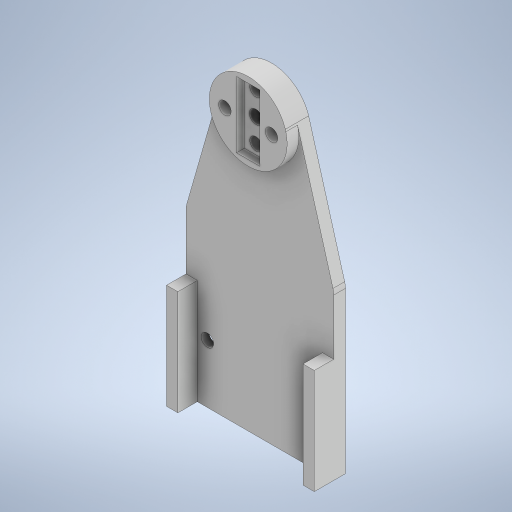
# Autodesk Inventor part: robot-arm-frame-output
Saved by Autodesk Inventor 2024.3 (Build 283343000, 343)
## iProperties
Created: 2024-11-17
Part Number: robot-arm-frame-output
Material: 一般
Document SubType Name: Modeling
Designer: azara
Density: 1 g/cm^3
Appearance: 既定
Author: azara
Autodesk Inventor part; units mm, degrees
ref_plane "YZ Plane" through (0, 0, 0) normal (1, 0, 0) x (0, 1, 0)
ref_plane "XZ Plane" through (0, 0, 0) normal (0, 1, 0) x (-1, 0, 0)
ref_plane "XY Plane" through (0, 0, 0) normal (0, 0, 1) x (1, 0, 0)
sketch "スケッチ1" plane through (0, 0, 0) normal (0, 0, 1) x (1, 0, 0)
  line L0 (0, 0) -> (38, 0)
  line L1 (38, 0) -> (38, 42)
  line L2 (38, 42) -> (0, 42)
  line L3 (0, 42) -> (0, 0)
  line L4 (19, 42) -> (19, 72)
  circle A0 centre (19, 72) radius 10
  line L5 (9.4606, 75) -> (28.5394, 75)
  line L6 (9.4606, 75) -> (0, 42)
  line L7 (28.5394, 75) -> (38, 42)
  dimension "d0" = 42
  dimension "d1" = 38
  dimension "d2" = 30
  dimension "d3" = 20
  dimension "d4" = 3
  constraints: 16 end point, 2 horizontal, 2 parallel, 2 point on circle, 1 centre point, 1 coincident, 1 midpoint, 1 perpendicular, 1 vertical
  measures "d0" distance of L0.end L1.end
  measures "d1" distance of L0.start L0.end
  measures "d2" distance of L4.start L4.end
  measures "d3" diameter of A0
  measures "d4" distance from line of L4.end L5
extrude "押し出し1" add sketch "スケッチ1" along normal blind 3
sketch "スケッチ2" plane through (0, 0, 3) normal (0, 0, 1) x (1, 0, 0)
  line L0 (0, 0) -> (38, 0) projected
  line L1 (38, 0) -> (38, 42) projected
  line L2 (38, 42) -> (28.5394, 75) projected
  arc A0 (28.5394, 75) -> (9.4606, 75) centre (19, 72) ccw projected
  circle A1 centre (19, 72) radius 10
  point P0 (9.4606, 75)
  point P1 (28.6799, 74.5099)
  constraints: 1 coincident, 3 other
extrude "押し出し2" add sketch "スケッチ2" along normal blind 3
sketch "スケッチ4" plane through (0, 0, 3) normal (0, 0, 1) x (1, 0, 0)
  line L0 (0, 42) -> (0, 0) projected
  line L1 (0, 0) -> (2.9, 0)
  line L2 (2.9, 0) -> (2.9, 27)
  line L3 (2.9, 27) -> (0, 27)
  line L4 (0, 27) -> (0, 0)
  line L5 (0, 0) -> (38, 0) projected
  line L6 (38, 0) -> (35.1, 0)
  line L7 (35.1, 0) -> (35.1, 27)
  line L8 (35.1, 27) -> (38, 27)
  line L9 (38, 27) -> (38, 0)
  point P0 (0, 27)
  dimension "d32" = 2.9
  dimension "d33" = 2.9
  dimension "d34" = 27
  dimension "d35" = 27
  constraints: 16 end point, 4 parallel, 2 horizontal, 2 perpendicular
  measures "d32" distance of L2.end L3.end
  measures "d33" distance of L7.end L8.end
  measures "d34" distance of L8.end L5.end
  measures "d35" distance of L1.end L2.end
extrude "押し出し3" add sketch "スケッチ4" along normal blind 5
sketch "スケッチ5" plane through (0, 0, 3) normal (0, 0, 1) x (1, 0, 0)
  line L0 (2.9, 0) -> (35.1, 0) projected
  line L1 (35.1, 27) -> (35.1, 0) projected
  point P0 (0, 0)
  point P1 (5.5, 15)
  point P2 (32.5, 15)
  dimension "d38" = 15
  dimension "d39" = 15
  dimension "d40" = 2.6
  dimension "d41" = 27
  measures "d38" distance from line of L0 point (32.5, 15)
  measures "d39" distance from line of L0 point (5.5, 15)
  measures "d40" distance from line of L1 point (32.5, 15)
  measures "d41" distance of point (32.5, 15) point (5.5, 15)
hole "穴2" at (5.5, 15, 3) at (32.5, 15, 3) direction (0, 0, -1) diameter 3.2 end through all
sketch "スケッチ7" plane through (0, 0, 0) normal (0, 0, -1) x (-1, 0, 0)
  circle A0 centre (-32.5, 15) radius 1.6 projected
  circle A1 centre (-32.5, 15) radius 4
  circle A2 centre (-5.5, 15) radius 1.6 projected
  circle A3 centre (-5.5, 15) radius 4
  point P0 (0, 0)
  dimension "d58" = 8
  dimension "d59" = 8
  constraints: 4 coincident, 2 centre point
  measures "d58" diameter of A1
  measures "d59" diameter of A3
extrude "押し出し4" cut sketch "スケッチ7" against normal blind 1
sketch "スケッチ8" plane through (0, 0, 0) normal (0, 0, -1) x (-1, 0, 0)
  circle A0 centre (-5.5, 15) radius 4 projected
  circle A1 centre (-32.5, 15) radius 4 projected
  line L0 (0, 42) -> (0, 0) projected
  line L1 (-9.4606, 75) -> (0, 42) projected
  arc A2 (-9.4606, 75) -> (-28.5394, 75) centre (-19, 72) ccw projected
  line L2 (-38, 42) -> (-28.5394, 75) projected
  line L3 (-38, 0) -> (-38, 42) projected
  line L4 (0, 0) -> (-38, 0) projected
  point P0 (-19, 78)
  point P1 (-25, 72)
  point P2 (-19, 66)
  point P3 (-13, 72)
  dimension "d62" = 6
  dimension "d65" = 360
  constraints: 5 other
  measures "d62" distance of A2.centre point (-19, 78)
hole "穴4" at (19, 78, 0) at (25, 72, 0) at (19, 66, 0) at (13, 72, 0) direction (0, 0, 1) diameter 3.2 end through all
sketch "スケッチ9" plane through (0, 0, 0) normal (0, 0, -1) x (-1, 0, 0)
  circle A0 centre (-13, 72) radius 1.6 projected
  circle A1 centre (-19, 66) radius 1.6 projected
  circle A2 centre (-25, 72) radius 1.6 projected
  circle A3 centre (-19, 78) radius 1.6 projected
  circle A4 centre (-5.5, 15) radius 4 projected
  circle A5 centre (-32.5, 15) radius 4 projected
  line L0 (0, 42) -> (0, 0) projected
  line L1 (-9.4606, 75) -> (0, 42) projected
  arc A6 (-9.4606, 75) -> (-28.5394, 75) centre (-19, 72) ccw projected
  line L2 (-38, 42) -> (-28.5394, 75) projected
  line L3 (-38, 0) -> (-38, 42) projected
  line L4 (0, 0) -> (-38, 0) projected
  constraints: 1 coincident
hole "穴5" at (19, 72, 0) direction (0, 0, 1) diameter 3.4 end through all
sketch "スケッチ10" plane through (0, 0, 6) normal (0, 0, 1) x (1, 0, 0)
  circle A0 centre (19, 72) radius 1.7 projected
  circle A1 centre (13, 72) radius 1.6 projected
  circle A2 centre (19, 66) radius 1.6 projected
  circle A3 centre (25, 72) radius 1.6 projected
  circle A4 centre (19, 78) radius 1.6 projected
  line L0 (28.6799, 74.5099) -> (28.5394, 75) projected
  arc A5 (28.5394, 75) -> (28.6799, 74.5099) centre (19, 72) ccw projected
  line L1 (16, 80.5) -> (22, 80.5)
  line L2 (22, 80.5) -> (22, 63.5)
  line L3 (22, 63.5) -> (16, 63.5)
  line L4 (16, 63.5) -> (16, 80.5)
  point P0 (0, 0)
  dimension "d81" = 8.5
  dimension "d82" = 17
  dimension "d83" = 6
  dimension "d84" = 3
  constraints: 8 end point, 2 parallel, 1 horizontal, 1 perpendicular
  measures "d81" distance from line of A0.centre L1
  measures "d82" distance of L3.end L1.start
  measures "d83" distance of L1.start L1.end
  measures "d84" distance from line of L2 A0.centre
extrude "押し出し5" cut sketch "スケッチ10" against normal blind 2 contours L1 L2 L3 L4
fillet "フィレット1" radius 5 2 edges at (38, 42, 1.5) (0, 42, 1.5)
